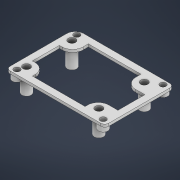
# Autodesk Inventor part: Adapter_Treiber
Saved by Autodesk Inventor 2021 (Build 250183000, 183)
## iProperties
Created: 2021-02-09
Part Number: Adapter_Treiber
Material: Generisch
Document SubType Name: Modeling
Designer: Ctroi
Density: 1 g/cm^3
Appearance: Vorgabe
Author: Ctroi
## iProperties of the stored document _3D-Druck.ipt
Created: 2021-02-09
Part Number: _3D-Druck
Material: Generisch
Document SubType Name: Modeling
Designer: Ctroi
Density: 1 g/cm^3
Appearance: Vorgabe
Author: Ctroi
Autodesk Inventor part; units mm, degrees
ref_plane "YZ Plane" through (0, 0, 0) normal (1, 0, 0) x (0, 1, 0)
ref_plane "XZ Plane" through (0, 0, 0) normal (0, 1, 0) x (-1, 0, 0)
ref_plane "XY Plane" through (0, 0, 0) normal (0, 0, 1) x (1, 0, 0)
sketch "Skizze1" plane through (0, 0, 0) normal (0, 1, 0) x (-1, 0, 0)
  line L0 (-37.5, 26.25) -> (37.5, 26.25)
  line L1 (37.5, 26.25) -> (37.5, -26.25)
  line L2 (37.5, -26.25) -> (-37.5, -26.25)
  line L3 (-37.5, -26.25) -> (-37.5, 26.25)
  line L4 (0, -36.75) -> (0, 36.75) projected
  line L5 (-52.5, 0) -> (52.5, 0) projected
  point P0 (0, 0)
  dimension "d0" = 75
  dimension "d1" = 52.5
  constraints: 8 end point, 2 parallel, 1 horizontal, 1 perpendicular, 2 other
  measures "d0" distance of L1.end L2.end
  measures "d1" distance of L0.end L1.end
extrude "Extrusion1" add sketch "Skizze1" along normal blind 2
sketch "Skizze2" plane through (0, 0, 0) normal (0, -1, 0) x (1, 0, 0)
  circle A0 centre (-31, 17.25) radius 3.5
  circle A1 centre (-31, -17.25) radius 3.5
  circle A2 centre (24, 17.25) radius 3.5
  circle A3 centre (24, -17.25) radius 3.5
  line L0 (-37.5, -26.25) -> (-37.5, 26.25) projected
  line L1 (-37.5, 26.25) -> (37.5, 26.25) projected
  line L2 (0, 37.1) -> (0, -37.1) projected
  line L3 (-52.5, 0) -> (52.5, 0) projected
  point P0 (0, 0)
  dimension "d4" = 7
  dimension "d5" = 7
  dimension "d6" = 7
  dimension "d7" = 7
  dimension "d8" = 34.5
  dimension "d12" = 17.25
  dimension "d13" = 17.25
  dimension "d14" = 34.5
  dimension "d15" = 55
  dimension "d16" = 31
  dimension "d17" = 31
  dimension "d18" = 55
  constraints: 4 centre point
  measures "d4" diameter of A0
  measures "d5" diameter of A1
  measures "d6" diameter of A2
  measures "d7" diameter of A3
  measures "d8" distance of A0.centre A1.centre
  measures "d12" distance from line of L3 A0.centre
  measures "d13" distance from line of L3 A2.centre
  measures "d14" distance of A2.centre A3.centre
  measures "d15" distance of A0.centre A2.centre
  measures "d16" distance from line of L2 A0.centre
  measures "d17" distance from line of L2 A1.centre
  measures "d18" distance of A1.centre A3.centre
extrude "Extrusion2" add sketch "Skizze2" along normal blind 15 contours A0 | A1 | A2 | A3
sketch "Skizze5" plane through (0, 2, 0) normal (0, 1, 0) x (1, 0, 0)
  circle A0 centre (-32.75, 22.75) radius 3.5
  circle A1 centre (32.75, 22.75) radius 3.5
  circle A2 centre (-32.75, -22.75) radius 3.5
  circle A3 centre (32.75, -22.75) radius 3.5
  line L0 (-37.5, -26.25) -> (37.5, -26.25) projected
  line L1 (-37.5, 26.25) -> (-37.5, -26.25) projected
  line L2 (37.5, 26.25) -> (-37.5, 26.25) projected
  circle A4 centre (-32.75, 22.75) radius 2.25
  circle A5 centre (-32.75, -22.75) radius 2.25
  circle A6 centre (32.75, -22.75) radius 2.25
  circle A7 centre (32.75, 22.75) radius 2.25
  line L3 (0, 37.1) -> (0, -37.1) projected
  line L4 (52.5, 0) -> (-52.5, 0) projected
  point P0 (0, 0)
  dimension "d33" = 7
  dimension "d34" = 7
  dimension "d35" = 7
  dimension "d36" = 7
  dimension "d39" = 65.5
  dimension "d40" = 4.75
  dimension "d42" = 45.5
  dimension "d44" = 65.5
  dimension "d45" = 4.5
  dimension "d46" = 4.5
  dimension "d47" = 4.5
  dimension "d48" = 4.5
  dimension "d66" = 22.75
  dimension "d67" = 32.75
  dimension "d68" = 32.75
  dimension "d69" = 22.75
  constraints: 8 centre point, 4 coincident
  measures "d33" diameter of A0
  measures "d34" diameter of A1
  measures "d35" diameter of A2
  measures "d36" diameter of A3
  measures "d39" distance of A3.centre A2.centre
  measures "d40" distance from line of L1 A2.centre
  measures "d42" distance of A2.centre A0.centre
  measures "d44" distance of A0.centre A1.centre
  measures "d45" diameter of A4
  measures "d46" diameter of A5
  measures "d47" diameter of A6
  measures "d48" diameter of A7
  measures "d66" distance from line of L4 A0.centre
  measures "d67" distance from line of L3 A0.centre
  measures "d68" distance from line of L3 A7.centre
  measures "d69" distance from line of L4 A3.centre
sketch "Skizze6" plane through (0, 0, 0) normal (0, -1, 0) x (1, 0, 0)
  circle A0 centre (32.75, -22.75) radius 3.5
  line L0 (37.5, -26.25) -> (-37.5, -26.25) projected
  line L1 (37.5, 26.25) -> (37.5, -26.25) projected
  circle A1 centre (32.75, 22.75) radius 3.5
  line L2 (-37.5, 26.25) -> (37.5, 26.25) projected
  circle A2 centre (-32.75, 22.75) radius 3.5
  line L3 (-37.5, -26.25) -> (-37.5, 26.25) projected
  circle A3 centre (-32.75, -22.75) radius 3.5
  line L4 (0, 37.1) -> (0, -37.1) projected
  line L5 (-52.5, 0) -> (52.5, 0) projected
  point P0 (0, 0)
  dimension "d50" = 7
  dimension "d53" = 7
  dimension "d56" = 7
  dimension "d59" = 7
  dimension "d70" = 32.75
  dimension "d71" = 22.75
  dimension "d72" = 32.75
  dimension "d73" = 32.75
  dimension "d74" = 22.75
  dimension "d75" = 32.75
  dimension "d76" = 22.75
  dimension "d103" = 3.5
  constraints: 4 centre point
  measures "d50" diameter of A0
  measures "d53" diameter of A1
  measures "d56" diameter of A2
  measures "d59" diameter of A3
  measures "d70" distance from line of L4 A1.centre
  measures "d71" distance from line of L5 A2.centre
  measures "d72" distance from line of L4 A2.centre
  measures "d73" distance from line of L4 A3.centre
  measures "d74" distance from line of L5 A3.centre
  measures "d75" distance from line of L4 A0.centre
  measures "d76" distance from line of L5 A0.centre
  measures "d103" distance from line of L2 A1.centre
extrude "Extrusion5" add sketch "Skizze6" along normal blind 4 contours A0 | A3 | A1 | A2
extrude "Extrusion6" cut sketch "Skizze5" against normal blind 6 contours A4 | A5 | A6 | A7
sketch "Skizze3" plane through (0, 2, 0) normal (0, 1, 0) x (1, 0, 0)
  circle A0 centre (-31, 17.25) radius 3.5 projected
  circle A1 centre (24, 17.25) radius 3.5 projected
  circle A2 centre (-31, -17.25) radius 3.5 projected
  circle A3 centre (24, -17.25) radius 3.5 projected
  circle A4 centre (-31, 17.25) radius 2.75
  circle A5 centre (24, 17.25) radius 2.75
  circle A6 centre (-31, -17.25) radius 2.75
  circle A7 centre (24, -17.25) radius 2.75
  point P0 (0, 0)
  dimension "d21" = 5.5
  dimension "d22" = 5.5
  dimension "d23" = 5.5
  dimension "d24" = 5.5
  constraints: 4 centre point, 4 coincident
  measures "d21" diameter of A4
  measures "d22" diameter of A5
  measures "d23" diameter of A6
  measures "d24" diameter of A7
extrude "Extrusion3" cut sketch "Skizze3" against normal blind 4 contours A4 | A5 | A6 | A7
sketch "Skizze4" plane through (24, -2, -17.25) normal (0, 1, 0) x (1, 0, 0)
  circle A0 centre (0, 0) radius 2.75 projected
  circle A1 centre (-55, 0) radius 2.75 projected
  circle A2 centre (-55, -34.5) radius 2.75 projected
  circle A3 centre (0, -34.5) radius 2.75 projected
  circle A4 centre (0, 0) radius 1.6
  circle A5 centre (-55, 0) radius 1.6
  circle A6 centre (-55, -34.5) radius 1.6
  circle A7 centre (0, -34.5) radius 1.6
  point P0 (-24, -17.25)
  dimension "d27" = 3.2
  dimension "d28" = 3.2
  dimension "d29" = 3.2
  dimension "d30" = 3.2
  constraints: 4 centre point, 4 coincident
  measures "d27" diameter of A4
  measures "d28" diameter of A5
  measures "d29" diameter of A6
  measures "d30" diameter of A7
extrude "Extrusion4" cut sketch "Skizze4" against normal up to surface (13 mm away) contours A4 | A5 | A6 | A7
sketch "Skizze7" plane through (0, 2, 0) normal (0, 1, 0) x (1, 0, 0)
  line L0 (-22.5, 21.25) -> (-22.5, 9.25)
  line L1 (-22.5, 9.25) -> (-32.5, 9.25)
  line L2 (-32.5, 9.25) -> (-32.5, -11.25)
  line L3 (-32.5, -11.25) -> (-22.5, -11.25)
  line L4 (-22.5, -11.25) -> (-22.5, -21.25)
  line L5 (-22.5, -21.25) -> (17.5, -21.25)
  line L6 (17.5, -21.25) -> (17.5, -11.25)
  line L7 (17.5, -11.25) -> (32.5, -11.25)
  line L8 (32.5, -11.25) -> (32.5, 9.25)
  line L9 (32.5, 9.25) -> (17.5, 9.25)
  line L10 (17.5, 9.25) -> (17.5, 21.25)
  line L11 (17.5, 21.25) -> (-22.5, 21.25)
  line L12 (-37.5, -26.25) -> (37.5, -26.25) projected
  line L13 (-37.5, 26.25) -> (-37.5, -26.25) projected
  line L14 (37.5, -26.25) -> (37.5, 26.25) projected
  line L15 (37.5, 26.25) -> (-37.5, 26.25) projected
  point P0 (0, 0)
  dimension "d77" = 5
  dimension "d78" = 5
  dimension "d79" = 15
  dimension "d80" = 15
  dimension "d83" = 5
  dimension "d84" = 15
  dimension "d86" = 17
  dimension "d87" = 17
  dimension "d88" = 5
  dimension "d89" = 5
  dimension "d93" = 17
  dimension "d94" = 5
  dimension "d95" = 17
  dimension "d96" = 20
  dimension "d97" = 20
  dimension "d98" = 5
  dimension "d99" = 15
  constraints: 24 end point, 2 parallel, 2 perpendicular, 1 point on line, 1 vertical
  measures "d77" distance from line of L12 L4.end
  measures "d78" distance from line of L12 L5.end
  measures "d79" distance from line of L13 L4.end
  measures "d80" distance from line of L13 L3.end
  measures "d83" distance from line of L13 L2.end
  measures "d84" distance from line of L12 L2.end
  measures "d86" distance from line of L15 L1.end
  measures "d87" distance from line of L15 L0.end
  measures "d88" distance from line of L15 L0.start
  measures "d89" distance from line of L15 L10.end
  measures "d93" distance from line of L15 L9.end
  measures "d94" distance between parallel lines of L14 L8
  measures "d95" distance between parallel lines of L15 L9
  measures "d96" distance between parallel lines of L14 L10
  measures "d97" distance between parallel lines of L14 L6
  measures "d98" distance from line of L14 L7.end
  measures "d99" distance from line of L12 L6.end
extrude "Extrusion7" cut sketch "Skizze7" against normal up to surface (2 mm away) contours L11 L10 L9 L8 L7 L6 L5 L4 L3 L2 L1 L0
fillet "Rundung1" radius 8 4 edges at (17.5, 1, -9.25) (-22.5, 1, -9.25) (17.5, 1, 11.25) (-22.5, 1, 11.25)
fillet "Rundung2" radius 6.5 1 edges at (-37.5, 1, -26.25)
fillet "Rundung3" radius 3 3 edges at (-37.5, 1, 26.25) (37.5, 1, 26.25) (37.5, 1, -26.25)
